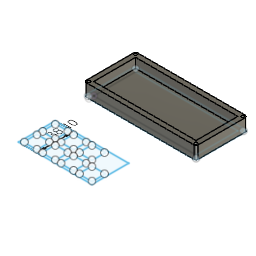
macrokitten (Autodesk Fusion 360 design; units mm, degrees)
Autodesk Fusion 360 part; units mm, degrees
sketch "Sketch1" plane through (0, 0, 0) normal (0, 0, 1) x (1, 0, 0)
  line L0 (0, 0) -> (106.2, 0)
  line L1 (106.2, 0) -> (106.2, 43.4)
  line L2 (106.2, 43.4) -> (0, 43.4)
  line L3 (0, 43.4) -> (0, 0)
  line L4 (-3, -5) -> (109.2, -5)
  line L5 (111.2, -3) -> (111.2, 46.4)
  line L6 (109.2, 48.4) -> (-3, 48.4)
  line L7 (-5, 46.4) -> (-5, -3)
  circle A0 centre (-2.55, 45.95) radius 1.45
  circle A1 centre (108.7, 45.9) radius 1.45
  arc A2 (-3, 48.4) -> (-5, 46.4) centre (-3, 46.4) ccw
  arc A3 (111.2, 46.4) -> (109.2, 48.4) centre (109.2, 46.4) ccw
  circle A4 centre (108.7, -2.5) radius 1.45
  arc A5 (109.2, -5) -> (111.2, -3) centre (109.2, -3) ccw
  line L8 (0, -5) -> (-0.4432, -4.5568) construction
  circle A6 centre (-2.5, -2.5) radius 1.45
  arc A7 (-5, -3) -> (-3, -5) centre (-3, -3) ccw
  dimension "d4" = 2.9
  dimension "d5" = 2.9
  dimension "d6" = 2
  dimension "d7" = 2
  dimension "d8" = 2.9
  dimension "d9" = 2
  dimension "d10" = 2.9
  dimension "d11" = 2
  constraint horizontal L0
  constraint vertical L1
  constraint horizontal L2
  constraint vertical L3
  constraint coincident L0.start L3.end
  constraint tangent L6 A2
  constraint tangent L7 A2
  constraint tangent L5 A3
  constraint tangent L6 A3
  constraint tangent L4 A5
  constraint tangent L5 A5
  constraint coincident L4 L8.start
  constraint tangent L4 A7
  constraint tangent L7 A7
  measures "d4" diameter of A0
  measures "d5" diameter of A1
  measures "d6" radius of A2
  measures "d7" radius of A3
  measures "d8" diameter of A4
  measures "d9" radius of A5
  measures "d10" diameter of A6
  measures "d11" radius of A7
extrude "Extrude1" add sketch "Sketch1" along normal blind 13 makes body 1
extrude "Extrude2" add sketch "Sketch1" along normal blind 3 separate body contours L0 L1 L2 L3 makes body 2
sketch "plate-2024-10-21T20_29_41.544Z" plane through (0, 0, 3) normal (0, 0, 1) x (1, 0, 0)
  line L0 (8.4683, -47.9448) -> (21.4683, -47.9448)
  line L1 (8.4683, -61.9448) -> (21.4683, -61.9448)
  line L2 (7.9683, -48.4448) -> (7.9683, -61.4448)
  line L3 (21.9683, -48.4448) -> (21.9683, -61.4448)
  arc A0 (8.4683, -47.9448) -> (7.9683, -48.4448) centre (8.4683, -48.4448) ccw
  arc A1 (21.9683, -48.4448) -> (21.4683, -47.9448) centre (21.4683, -48.4448) ccw
  arc A2 (7.9683, -61.4448) -> (8.4683, -61.9448) centre (8.4683, -61.4448) ccw
  arc A3 (21.4683, -61.9448) -> (21.9683, -61.4448) centre (21.4683, -61.4448) ccw
  line L4 (27.5183, -47.9448) -> (40.5183, -47.9448)
  line L5 (27.5183, -61.9448) -> (40.5183, -61.9448)
  line L6 (27.0183, -48.4448) -> (27.0183, -61.4448)
  line L7 (41.0183, -48.4448) -> (41.0183, -61.4448)
  arc A4 (27.5183, -47.9448) -> (27.0183, -48.4448) centre (27.5183, -48.4448) ccw
  arc A5 (41.0183, -48.4448) -> (40.5183, -47.9448) centre (40.5183, -48.4448) ccw
  arc A6 (27.0183, -61.4448) -> (27.5183, -61.9448) centre (27.5183, -61.4448) ccw
  arc A7 (40.5183, -61.9448) -> (41.0183, -61.4448) centre (40.5183, -61.4448) ccw
  line L8 (46.5683, -47.9448) -> (59.5683, -47.9448)
  line L9 (46.5683, -61.9448) -> (59.5683, -61.9448)
  line L10 (46.0683, -48.4448) -> (46.0683, -61.4448)
  line L11 (60.0683, -48.4448) -> (60.0683, -61.4448)
  arc A8 (46.5683, -47.9448) -> (46.0683, -48.4448) centre (46.5683, -48.4448) ccw
  arc A9 (60.0683, -48.4448) -> (59.5683, -47.9448) centre (59.5683, -48.4448) ccw
  arc A10 (46.0683, -61.4448) -> (46.5683, -61.9448) centre (46.5683, -61.4448) ccw
  arc A11 (59.5683, -61.9448) -> (60.0683, -61.4448) centre (59.5683, -61.4448) ccw
  line L12 (8.4683, -66.9948) -> (21.4683, -66.9948)
  line L13 (8.4683, -80.9948) -> (21.4683, -80.9948)
  line L14 (7.9683, -67.4948) -> (7.9683, -80.4948)
  line L15 (21.9683, -67.4948) -> (21.9683, -80.4948)
  arc A12 (8.4683, -66.9948) -> (7.9683, -67.4948) centre (8.4683, -67.4948) ccw
  arc A13 (21.9683, -67.4948) -> (21.4683, -66.9948) centre (21.4683, -67.4948) ccw
  arc A14 (7.9683, -80.4948) -> (8.4683, -80.9948) centre (8.4683, -80.4948) ccw
  arc A15 (21.4683, -80.9948) -> (21.9683, -80.4948) centre (21.4683, -80.4948) ccw
  line L16 (27.5183, -66.9948) -> (40.5183, -66.9948)
  line L17 (27.5183, -80.9948) -> (40.5183, -80.9948)
  line L18 (27.0183, -67.4948) -> (27.0183, -80.4948)
  line L19 (41.0183, -67.4948) -> (41.0183, -80.4948)
  arc A16 (27.5183, -66.9948) -> (27.0183, -67.4948) centre (27.5183, -67.4948) ccw
  arc A17 (41.0183, -67.4948) -> (40.5183, -66.9948) centre (40.5183, -67.4948) ccw
  arc A18 (27.0183, -80.4948) -> (27.5183, -80.9948) centre (27.5183, -80.4948) ccw
  arc A19 (40.5183, -80.9948) -> (41.0183, -80.4948) centre (40.5183, -80.4948) ccw
  line L20 (46.5683, -66.9948) -> (59.5683, -66.9948)
  line L21 (46.5683, -80.9948) -> (59.5683, -80.9948)
  line L22 (46.0683, -67.4948) -> (46.0683, -80.4948)
  line L23 (60.0683, -67.4948) -> (60.0683, -80.4948)
  arc A20 (46.5683, -66.9948) -> (46.0683, -67.4948) centre (46.5683, -67.4948) ccw
  arc A21 (60.0683, -67.4948) -> (59.5683, -66.9948) centre (59.5683, -67.4948) ccw
  arc A22 (46.0683, -80.4948) -> (46.5683, -80.9948) centre (46.5683, -80.4948) ccw
  arc A23 (59.5683, -80.9948) -> (60.0683, -80.4948) centre (59.5683, -80.4948) ccw
  line L24 (65.6183, -66.9948) -> (78.6183, -66.9948)
  line L25 (65.6183, -80.9948) -> (78.6183, -80.9948)
  line L26 (65.1183, -67.4948) -> (65.1183, -80.4948)
  line L27 (79.1183, -67.4948) -> (79.1183, -80.4948)
  arc A24 (65.6183, -66.9948) -> (65.1183, -67.4948) centre (65.6183, -67.4948) ccw
  arc A25 (79.1183, -67.4948) -> (78.6183, -66.9948) centre (78.6183, -67.4948) ccw
  arc A26 (65.1183, -80.4948) -> (65.6183, -80.9948) centre (65.6183, -80.4948) ccw
  arc A27 (78.6183, -80.9948) -> (79.1183, -80.4948) centre (78.6183, -80.4948) ccw
  line L28 (5.4433, -83.5198) -> (81.6433, -83.5198)
  line L29 (5.4433, -45.4198) -> (81.6433, -45.4198)
  line L30 (5.4433, -83.5198) -> (5.4433, -45.4198)
  line L31 (81.6433, -83.5198) -> (81.6433, -45.4198)
  dimension "d16" = 38.1
  measures "d16" distance of L28.start L29.start
